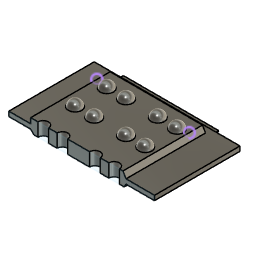
Rivets_Model_Double riveted, double strap chain butt joint (Autodesk Fusion 360 design; units mm, degrees)
Autodesk Fusion 360 part; units mm, degrees
note: some values were not read from the file. Set by a fixed rule: which sketch regions a step uses.
sketch "Sketch1" plane through (0, 0, 0) normal (0, 1, 0) x (1, 0, 0)
  line L0 (0, -3.5) -> (115, -3.5)
  line L1 (115, -3.5) -> (115, 0)
  line L2 (-105, 0) -> (-105, -3.5)
  line L3 (-105, -3.5) -> (-17, -3.5)
  line L4 (-17, -3.5) -> (-14.5, -3.5)
  line L5 (-14.5, -3.5) -> (0, -3.5)
  line L6 (-105, 0) -> (-105, 3.5)
  line L7 (-105, 3.5) -> (115, 3.5)
  line L8 (115, 3.5) -> (115, 0)
  line L9 (0, 3.5) -> (-72, 3.5)
  line L10 (0, 3.5) -> (72, 3.5)
  line L11 (0, 8.5) -> (-66.8485, 8.5)
  line L12 (-66.8485, 8.5) -> (69.1132, 8.5)
  line L13 (0, -11.5) -> (-72, -11.5)
  line L14 (-72, -11.5) -> (67.3812, -11.5)
  line L15 (0, -3.5) -> (-72, -3.5)
  line L16 (0, -3.5) -> (72, -3.5)
  line L17 (-72, -3.5) -> (-72, -11.5)
  line L18 (72, -3.5) -> (67.3812, -11.5)
  line L19 (72, -3.5) -> (96.1714, -3.5) construction
  line L20 (-72, 3.5) -> (-66.8485, 8.5)
  line L21 (72, 3.5) -> (69.1132, 8.5)
  line L22 (72, 3.5) -> (49.3136, 3.5) construction
  dimension "d1" = 3.5
  dimension "d2" = 3.5
  dimension "d3" = 72
  dimension "d4" = 72
  dimension "d5" = 5
  dimension "d6" = 8
  dimension "d7" = 72
  dimension "d8" = 72
  dimension "d9" = 120
  dimension "d11" = 60
  constraint perpendicular L0 L1
  constraint perpendicular L2 L3
  constraint parallel L3 L4
  constraint perpendicular L6 L7
  constraint coincident L7 L9.start
  constraint perpendicular L14 L17
  constraint horizontal L19
  constraint horizontal L22
  measures "d1" distance of origin L0.start
  measures "d2" distance of L2.start L6.end
  measures "d3" distance of L9.start L9.end
  measures "d4" distance of L9.start L10.end
  measures "d5" distance of L9.start L11.start
  measures "d6" distance of L0.start L13.start
  measures "d7" distance of L0.start L15.end
  measures "d8" distance of L0.start L16.end
  measures "d9" angle of L18 L19
  measures "d11" angle of L21 L22
extrude "Extrude1" add sketch "Sketch1" along normal mid plane 100 makes body 1
sketch "Sketch2" plane through (0, -50, 0) normal (0, -1, 0) x (1, 0, 0)
  line L0 (72, -3.5) -> (115, -3.5)
  line L1 (115, -3.5) -> (115, 3.5)
  line L2 (115, 3.5) -> (72, 3.5)
  line L3 (72, 3.5) -> (67.3812, 11.5)
  line L4 (67.3812, 11.5) -> (-72, 11.5)
  line L5 (-72, 11.5) -> (-72, 3.5)
  line L6 (-72, 3.5) -> (-105, 3.5)
  line L7 (-105, 3.5) -> (-105, -3.5)
  line L8 (-105, -3.5) -> (-72, -3.5)
  line L9 (-72, -3.5) -> (-66.8485, -8.5)
  line L10 (-66.8485, -8.5) -> (69.1132, -8.5)
  line L11 (69.1132, -8.5) -> (72, -3.5)
sketch "Sketch3" plane through (0, 0, 11.5) normal (0, 0, 1) x (-1, 0, 0)
  line L0 (-67.3812, 50) -> (-67.3812, -50)
  line L1 (72, -50) -> (72, 50)
  line L2 (72, 50) -> (-67.3812, 50)
sketch "Sketch4" plane through (0, 50, 0) normal (0, 1, 0) x (-1, 0, 0)
  line L0 (-115, -3.5) -> (-72, -3.5)
  line L1 (-72, -3.5) -> (-69.1132, -8.5)
  line L2 (-69.1132, -8.5) -> (66.8485, -8.5)
  line L3 (66.8485, -8.5) -> (72, -3.5)
  line L4 (72, -3.5) -> (105, -3.5)
  line L5 (105, -3.5) -> (105, 3.5)
  line L6 (105, 3.5) -> (72, 3.5)
  line L7 (72, 3.5) -> (72, 11.5)
  line L8 (72, 11.5) -> (-67.3812, 11.5)
  line L9 (-67.3812, 11.5) -> (-72, 3.5)
  line L10 (-72, 3.5) -> (-115, 3.5)
  line L11 (-115, 3.5) -> (-115, -3.5)
  line L12 (-72, 3.5) -> (72, 3.5)
  line L13 (-72, 3.5) -> (-67.3812, 11.5)
  line L14 (-67.3812, 11.5) -> (72, 11.5)
  line L15 (-72, -3.5) -> (-69.1132, -8.5)
  line L16 (-69.1132, -8.5) -> (66.8485, -8.5)
  line L17 (66.8485, -8.5) -> (72, -3.5)
  line L18 (-72, -3.5) -> (72, -3.5)
  line L19 (-72, 3.5) -> (-115, 3.5)
  line L20 (-115, 3.5) -> (-115, -3.5)
  line L21 (-115, -3.5) -> (105, -3.5)
  line L22 (105, 3.5) -> (72, 3.5)
  constraint coincident L9.end L10.start
  constraint coincident L6.end L7.start
  constraint coincident L8.end L9.start
  constraint coincident L7.end L8.start
  constraint coincident L0.end L1.start
  constraint coincident L1.end L2.start
  constraint coincident L2.end L3.start
  constraint coincident L3.end L4.start
  constraint coincident L10.end L11.start
  constraint coincident L0.start L11.end
  constraint coincident L4.end L5.start
  constraint coincident L5.end L6.start
extrude "Extrude2" add sketch "Sketch4" along normal blind 25 contours L1 L2 L3 L15 L16 L17 L18 L21 bodies 1
sketch "Sketch5" plane through (0, 50, 0) normal (0, 1, 0) x (-1, 0, 0)
  line L0 (-72, -3.5) -> (72, -3.5)
  line L1 (72, -3.5) -> (105, -3.5)
  line L2 (105, -3.5) -> (105, 3.5)
  line L3 (105, 3.5) -> (72, 3.5)
  line L4 (72, 3.5) -> (72, 11.5)
  line L5 (72, 11.5) -> (-67.3812, 11.5)
  line L6 (-67.3812, 11.5) -> (-72, 3.5)
  line L7 (-72, 3.5) -> (-115, 3.5)
  line L8 (-115, 3.5) -> (-115, -3.5)
  line L9 (-115, -3.5) -> (-72, -3.5)
  line L10 (-72, 3.5) -> (72, 3.5)
  line L11 (72, 3.5) -> (105, 3.5)
  line L12 (105, 3.5) -> (105, -3.5)
  line L13 (-72, 3.5) -> (-115, 3.5)
  line L14 (-115, 3.5) -> (-115, -3.5)
  line L15 (-115, -3.5) -> (105, -3.5)
  constraint coincident L6.end L7.start
  constraint coincident L3.end L4.start
  constraint coincident L2.end L3.start
  constraint coincident L1.end L2.start
  constraint coincident L7.end L8.start
  constraint coincident L8.end L9.start
extrude "Extrude3" add sketch "Sketch5" along normal blind 17 contours L0 L1 L2 L3 L7 L8 L9 L10 L11 L12 L13 L14 L15 bodies 1
sketch "Sketch6" plane through (0, 50, 0) normal (0, 1, 0) x (-1, 0, 0)
  line L0 (-72, 3.5) -> (72, 3.5)
  line L1 (72, 3.5) -> (72, 11.5)
  line L2 (72, 11.5) -> (-67.3812, 11.5)
  line L3 (-67.3812, 11.5) -> (-72, 3.5)
sketch "Sketch7" plane through (0, 0, 11.5) normal (0, 0, 1) x (-1, 0, 0)
sketch "Sketch8" plane through (0, 0, 11.5) normal (0, 0, 1) x (-1, 0, 0)
  line L0 (0, -50) -> (0, 50)
  line L1 (0, 50) -> (0, 0)
  line L2 (24, 50) -> (24, -50)
  line L3 (-25, 0) -> (-25, -50)
  line L4 (-25, -50) -> (-25, 50)
  line L5 (-25, 50) -> (-25, 0)
  line L6 (-54, 50) -> (-54, -50)
  circle A0 centre (53, 50) radius 8
  circle A1 centre (24, 50) radius 8
  circle A2 centre (-25, 50) radius 8
  circle A3 centre (-54, 50) radius 8
  line L7 (53, 50) -> (53, 2)
  dimension "d22" = 29
  dimension "d23" = 29
  dimension "d24" = 16
  dimension "d25" = 16
  dimension "d26" = 16
  dimension "d27" = 16
  dimension "d28" = 48
  constraint vertical L0
  constraint coincident L1.end origin
  constraint parallel L0 L1
  constraint coincident L2.start A1.centre
  constraint coincident L4.end L5.start
  constraint coincident L6.start A3.centre
  constraint coincident A0.centre L7.start
  measures "d22" distance of L2.start A0.centre
  measures "d23" distance of L4.end L6.start
  measures "d24" diameter of A0
  measures "d25" diameter of A1
  measures "d26" diameter of A2
  measures "d27" diameter of A3
  measures "d28" distance of A0.centre L7.end
sketch "Sketch9" plane through (0, 50, 0) normal (0, 1, 0) x (-1, 0, 0)
extrude "Extrude4" add 1 faces at (-22.2828, 75, -5.1667) along direction (0, 1, 0) blind 15 on bodies 1 bodies 1
extrude "Extrude5" add 1 faces at (27.3333, 67, 1.1667) along direction (0, 1, 0) blind 12 on bodies 1 bodies 1
extrude "Extrude6" add sketch "Sketch6" along normal blind 20 bodies 1
sketch "Sketch10" plane through (0, 0, 0) normal (0, 1, 0) x (1, 0, 0)
sketch "Sketch11" plane through (0, 0, 11.5) normal (0, 0, 1) x (-1, 0, 0)
sketch "Sketch12" plane through (0, 0, 11.5) normal (0, 0, 1) x (1, 0, 0)
sketch "Sketch13" plane through (0, 0, 11.5) normal (0, 0, 1) x (-1, 0, 0)
sketch "Sketch14" plane through (0, 0, 11.5) normal (0, 0, 1) x (1, 0, 0)
sketch "Sketch15" plane through (0, 0, 11.5) normal (0, 0, 1) x (-1, 0, 0)
ref_plane "WorkPlane1" through (67.3812, 70, 11.5) normal (0, 0, 1) x (1, 0, 0)
sketch "Sketch16" plane through (0, 0, 11.5) normal (0, 0, 1) x (1, 0, 0)
  line L0 (0, 0) -> (0, -50)
  line L1 (0, -50) -> (-24, -50)
  line L2 (0, -50) -> (24, -50)
  line L3 (-24, 70) -> (-24, -50)
  circle A0 centre (-53, -2) radius 8
  circle A1 centre (-53, 46) radius 8
  circle A2 centre (24, -2) radius 8
  circle A3 centre (24, 46) radius 8
  circle A4 centre (53, -2) radius 8
  circle A5 centre (53, 46) radius 8
  line L4 (53, -50) -> (66.9727, -50)
  arc A6 (-45, -50) -> (-61, -50) centre (-53, -50) ccw
  arc A7 (-16, -50) -> (-24, -42) centre (-24, -50) ccw
  arc A8 (32, -50) -> (16, -50) centre (24, -50) ccw
  arc A9 (61, -50) -> (45, -50) centre (53, -50) ccw
  line L5 (0, -50) -> (53, -50)
  line L6 (-45, -50) -> (-24, -50)
  line L7 (-16, -50) -> (66.9727, -50)
  line L8 (-24, -50) -> (-24, -2)
  circle A10 centre (-24, -2) radius 8
  line L9 (-24, -2) -> (-24, 46)
  circle A11 centre (-24, 46) radius 8
  dimension "d36" = 24
  dimension "d37" = 29
  dimension "d38" = 24
  dimension "d39" = 29
  dimension "d41" = 16
  dimension "d42" = 16
  dimension "d43" = 16
  dimension "d44" = 16
  dimension "d45" = 48
  dimension "d46" = 16
  dimension "d47" = 48
  dimension "d48" = 16
  dimension "d49" = 48
  dimension "d50" = 16
  dimension "d51" = 48
  dimension "d52" = 16
  dimension "d53" = 48
  dimension "d54" = 16
  dimension "d55" = 48
  dimension "d56" = 16
  dimension "d57" = 48
  dimension "d58" = 16
  dimension "d59" = 48
  dimension "d60" = 16
  constraint coincident L0.start origin
  constraint vertical L0
  constraint perpendicular L0 L1
  constraint perpendicular L0 L2
  constraint perpendicular L1 L3
  constraint coincident L1.end L3.end
  constraint coincident L2.end A8.centre
  constraint coincident L4.start A9.centre
  constraint parallel L2 L4
  constraint coincident L1 A7.start
  constraint coincident L2 A8.end
  constraint coincident L4 A9.start
  constraint collinear L6 L7
  constraint coincident L3 A7.end
  constraint perpendicular L1 L8
  constraint coincident L8.end A10.centre
  constraint parallel L3 L9
  constraint coincident L9.end A11.centre
  measures "d36" distance of L0.end L1.end
  measures "d37" distance of L1.end A6.centre
  measures "d38" distance of L0.end L2.end
  measures "d39" distance of L2.end L4.start
  measures "d41" diameter of A6
  measures "d42" diameter of A7
  measures "d43" diameter of A8
  measures "d44" diameter of A9
  measures "d45" distance of A6.centre A0.centre
  measures "d46" diameter of A0
  measures "d47" distance of A0.centre A1.centre
  measures "d48" diameter of A1
  measures "d49" distance of L2.end A2.centre
  measures "d50" diameter of A2
  measures "d51" distance of A2.centre A3.centre
  measures "d52" diameter of A3
  measures "d53" distance of L4.start A4.centre
  measures "d54" diameter of A4
  measures "d55" distance of A4.centre A5.centre
  measures "d56" diameter of A5
  measures "d57" distance of L1.end L8.end
  measures "d58" diameter of A10
  measures "d59" distance of L8.end L9.end
  measures "d60" diameter of A11
extrude "Extrude7" cut sketch "Sketch16" sketch "Sketch8" against normal blind 200 contours L3 L9 A11 | L3 L9 A11 | L3 L8 A10 L9 | L3 L8 A10 L9 | A0 | A1 | A2 | A3 | A4 | A5 of sketch 2 bodies 1
sketch "Sketch17" plane through (0, -50, 0) normal (0, -1, 0) x (1, 0, 0)
  line L0 (-152, 6) -> (-144, 6)
  line L1 (-144, 6) -> (-144, -4)
  line L2 (-152, -4) -> (-152, 6)
  line L3 (-152, 6) -> (-142, 6)
  line L4 (-152, 6) -> (-152, 16)
  line L5 (-152, 6) -> (-142, 6) construction
  arc A0 (-142, 6) -> (-152, 16) centre (-152, 6) ccw
  line L6 (-152, -14) -> (-152, -24)
  arc A1 (-152, -24) -> (-142, -14) centre (-152, -14) ccw
  line L7 (-152, -14) -> (-144, -14)
  line L8 (-152, -4) -> (-152, -14)
  line L9 (-144, -14) -> (-144, -4)
  line L10 (-152, -14) -> (-142, -14) construction
  line L11 (-144, -14) -> (-142, -14)
  dimension "d63" = 8
  dimension "d64" = 10
  dimension "d65" = 10
  dimension "d66" = 10
  constraint horizontal L0
  constraint vertical L1
  constraint vertical L2
  constraint perpendicular L2 L3
  constraint perpendicular L3 L4
  constraint horizontal L5
  measures "d63" distance of L0.start L0.end
  measures "d64" distance of L0.start L2.start
  measures "d65" distance of L0.start L3.end
  measures "d66" distance of L0.start L4.end
revolve "Revolve1" add sketch "Sketch17" angle 360 about axis through (-152, -50, -4) along (0, 0, 1) separate body makes body 2
copy_body "CopyPasteBodies1" bodies 2 makes body 3
move_body "Move1" bodies 3 to x (1, 0, 0) y (0, 1, 0) z (0, 0, 1) at (99, 48, 5.5)
copy_body "CopyPasteBodies2" bodies 2 makes body 4
move_body "Move2" bodies 4 to x (1, 0, 0) y (0, 1, 0) z (0, 0, 1) at (128, 48, 5.5)
copy_body "CopyPasteBodies3" bodies 2 makes body 5
move_body "Move3" bodies 5 to x (1, 0, 0) y (0, 1, 0) z (0, 0, 1) at (176, 48, 5.5)
copy_body "CopyPasteBodies4" bodies 2 makes body 6
move_body "Move4" bodies 6 to x (1, 0, 0) y (0, 1, 0) z (0, 0, 1) at (99, 96, 5.5)
copy_body "CopyPasteBodies5" bodies 2 makes body 7
move_body "Move5" bodies 7 to x (1, 0, 0) y (0, 1, 0) z (0, 0, 1) at (205, 48, 5.5)
copy_body "CopyPasteBodies6" bodies 2 makes body 8
move_body "Move6" bodies 8 to x (1, 0, 0) y (0, 1, 0) z (0, 0, 1) at (128, 96, 5.5)
copy_body "CopyPasteBodies7" bodies 2 makes body 9
move_body "Move7" bodies 9 to x (1, 0, 0) y (0, 1, 0) z (0, 0, 1) at (176, 96, 5.5)
move_body "Move8" bodies 2 to x (1, 0, 0) y (0, 1, 0) z (0, 0, 1) at (205, 96, 5.5)
